Autodesk Fusion 360 part; units mm, degrees
note: some values were not read from the file. Chosen so that the rebuilt part matches the saved one: which pieces of a blend or face edit are solid. Set by a fixed rule: which sketch regions a step uses.
(part 2 of 3)
  line L805 (266.727767, 11.986044) -> (273.65597, -0.013956)
  line L806 (273.65597, -0.013956) -> (287.512376, -0.013956)
  line L807 (287.512376, -0.013956) -> (294.44058, 11.986044)
  line L808 (294.44058, 11.986044) -> (287.512376, 23.986044)
  line L809 (290.110453, 25.486044) -> (297.038656, 13.486044)
  line L810 (297.038656, 37.486044) -> (290.110453, 25.486044)
  line L811 (310.895062, 37.486044) -> (297.038656, 37.486044)
  line L812 (317.823265, 25.486044) -> (310.895062, 37.486044)
  line L813 (310.895062, 13.486044) -> (317.823265, 25.486044)
  line L814 (320.421342, 23.986044) -> (313.493138, 11.986044)
  line L815 (297.038656, 13.486044) -> (310.895062, 13.486044)
  line L816 (310.895062, 10.486044) -> (297.038656, 10.486044)
  line L817 (317.823265, -1.513956) -> (310.895062, 10.486044)
  line L818 (310.895062, -13.513956) -> (317.823265, -1.513956)
  line L819 (297.038656, -13.513956) -> (310.895062, -13.513956)
  line L820 (290.110453, -1.513956) -> (297.038656, -13.513956)
  line L821 (297.038656, 10.486044) -> (290.110453, -1.513956)
  line L822 (334.277748, 23.986044) -> (320.421342, 23.986044)
  line L823 (313.493138, 11.986044) -> (320.421342, -0.013956)
  line L824 (320.421342, -0.013956) -> (334.277748, -0.013956)
  line L825 (334.277748, -0.013956) -> (341.205951, 11.986044)
  line L826 (341.205951, 11.986044) -> (334.277748, 23.986044)
  line L827 (334.277748, -3.013956) -> (320.421342, -3.013956)
  line L828 (320.421342, -3.013956) -> (313.493138, -15.013956)
  line L829 (313.493138, -15.013956) -> (320.421342, -27.013956)
  line L830 (320.421342, -27.013956) -> (334.277748, -27.013956)
  line L831 (334.277748, -27.013956) -> (341.205951, -15.013956)
  line L832 (341.205951, -15.013956) -> (334.277748, -3.013956)
  line L833 (336.875824, -1.513956) -> (343.804028, -13.513956)
  line L834 (343.804028, 10.486044) -> (336.875824, -1.513956)
  line L835 (357.660434, 10.486044) -> (343.804028, 10.486044)
  line L836 (364.588637, -1.513956) -> (357.660434, 10.486044)
  line L837 (357.660434, -13.513956) -> (364.588637, -1.513956)
  line L838 (367.186713, -3.013956) -> (360.25851, -15.013956)
  line L839 (343.804028, -13.513956) -> (357.660434, -13.513956)
  line L840 (357.660434, -16.513956) -> (343.804028, -16.513956)
  line L841 (364.588637, -28.513956) -> (357.660434, -16.513956)
  line L842 (357.660434, -40.513956) -> (364.588637, -28.513956)
  line L843 (343.804028, -40.513956) -> (357.660434, -40.513956)
  line L844 (336.875824, -28.513956) -> (343.804028, -40.513956)
  line L845 (343.804028, -16.513956) -> (336.875824, -28.513956)
  line L846 (381.04312, -3.013956) -> (367.186713, -3.013956)
  line L847 (360.25851, -15.013956) -> (367.186713, -27.013956)
  line L848 (367.186713, -27.013956) -> (381.04312, -27.013956)
  line L849 (381.04312, -27.013956) -> (387.971323, -15.013956)
  line L850 (387.971323, -15.013956) -> (381.04312, -3.013956)
  line L851 (381.04312, -30.013956) -> (367.186713, -30.013956)
  line L852 (367.186713, -30.013956) -> (360.25851, -42.013956)
  line L853 (360.25851, -42.013956) -> (367.186713, -54.013956)
  line L854 (367.186713, -54.013956) -> (381.04312, -54.013956)
  line L855 (381.04312, -54.013956) -> (387.971323, -42.013956)
  line L856 (387.971323, -42.013956) -> (381.04312, -30.013956)
  line L857 (383.641196, -28.513956) -> (390.569399, -40.513956)
  line L858 (390.569399, -16.513956) -> (383.641196, -28.513956)
  line L859 (404.425806, -16.513956) -> (390.569399, -16.513956)
  line L860 (411.354009, -28.513956) -> (404.425806, -16.513956)
  line L861 (404.425806, -40.513956) -> (411.354009, -28.513956)
  line L862 (413.952085, -30.013956) -> (407.023882, -42.013956)
  line L863 (390.569399, -40.513956) -> (404.425806, -40.513956)
  line L864 (404.425806, -43.513956) -> (390.569399, -43.513956)
  line L865 (411.354009, -55.513956) -> (404.425806, -43.513956)
  line L866 (404.425806, -67.513956) -> (411.354009, -55.513956)
  line L867 (390.569399, -67.513956) -> (404.425806, -67.513956)
  line L868 (383.641196, -55.513956) -> (390.569399, -67.513956)
  line L869 (390.569399, -43.513956) -> (383.641196, -55.513956)
  line L870 (427.808492, -30.013956) -> (413.952085, -30.013956)
  line L871 (407.023882, -42.013956) -> (413.952085, -54.013956)
  line L872 (413.952085, -54.013956) -> (427.808492, -54.013956)
  line L873 (427.808492, -54.013956) -> (434.736695, -42.013956)
  line L874 (434.736695, -42.013956) -> (427.808492, -30.013956)
  line L875 (427.808492, -57.013956) -> (413.952085, -57.013956)
  line L876 (413.952085, -57.013956) -> (407.023882, -69.013956)
  line L877 (407.023882, -69.013956) -> (413.952085, -81.013956)
  line L878 (413.952085, -81.013956) -> (427.808492, -81.013956)
  line L879 (427.808492, -81.013956) -> (434.736695, -69.013956)
  line L880 (434.736695, -69.013956) -> (427.808492, -57.013956)
  line L881 (430.406568, -55.513956) -> (437.334771, -67.513956)
  line L882 (437.334771, -43.513956) -> (430.406568, -55.513956)
  line L883 (451.191178, -43.513956) -> (437.334771, -43.513956)
  line L884 (458.119381, -55.513956) -> (451.191178, -43.513956)
  line L885 (451.191178, -67.513956) -> (458.119381, -55.513956)
  line L886 (460.717457, -57.013956) -> (453.789254, -69.013956)
  line L887 (437.334771, -67.513956) -> (451.191178, -67.513956)
  line L888 (451.191178, -70.513956) -> (437.334771, -70.513956)
  line L889 (458.119381, -82.513956) -> (451.191178, -70.513956)
  line L890 (451.191178, -94.513956) -> (458.119381, -82.513956)
  line L891 (437.334771, -94.513956) -> (451.191178, -94.513956)
  line L892 (430.406568, -82.513956) -> (437.334771, -94.513956)
  line L893 (437.334771, -70.513956) -> (430.406568, -82.513956)
  line L894 (474.573864, -57.013956) -> (460.717457, -57.013956)
  line L895 (453.789254, -69.013956) -> (460.717457, -81.013956)
  line L896 (460.717457, -81.013956) -> (474.573864, -81.013956)
  line L897 (474.573864, -81.013956) -> (481.502067, -69.013956)
  line L898 (481.502067, -69.013956) -> (474.573864, -57.013956)
  line L899 (474.573864, -84.013956) -> (460.717457, -84.013956)
  line L900 (460.717457, -84.013956) -> (453.789254, -96.013956)
  line L901 (453.789254, -96.013956) -> (460.717457, -108.013956)
  line L902 (460.717457, -108.013956) -> (474.573864, -108.013956)
  line L903 (474.573864, -108.013956) -> (481.502067, -96.013956)
  line L904 (481.502067, -96.013956) -> (474.573864, -84.013956)
  line L905 (79.663594, 200.981392) -> (86.591797, 188.981392)
  line L906 (86.591797, 212.981392) -> (79.663594, 200.981392)
  line L907 (100.448203, 212.981392) -> (86.591797, 212.981392)
  line L908 (107.376406, 200.981392) -> (100.448203, 212.981392)
  line L909 (100.448203, 188.981392) -> (107.376406, 200.981392)
  line L910 (109.974483, 199.481392) -> (103.046279, 187.481392)
  line L911 (86.591797, 188.981392) -> (100.448203, 188.981392)
  line L912 (100.448203, 185.981392) -> (86.591797, 185.981392)
  line L913 (107.376406, 173.981392) -> (100.448203, 185.981392)
  line L914 (100.448203, 161.981392) -> (107.376406, 173.981392)
  line L915 (86.591797, 161.981392) -> (100.448203, 161.981392)
  line L916 (79.663594, 173.981392) -> (86.591797, 161.981392)
  line L917 (86.591797, 185.981392) -> (79.663594, 173.981392)
  line L918 (123.830889, 199.481392) -> (109.974483, 199.481392)
  line L919 (103.046279, 187.481392) -> (109.974483, 175.481392)
  line L920 (109.974483, 175.481392) -> (123.830889, 175.481392)
  line L921 (123.830889, 175.481392) -> (130.759092, 187.481392)
  line L922 (130.759092, 187.481392) -> (123.830889, 199.481392)
  line L923 (123.830889, 172.481392) -> (109.974483, 172.481392)
  line L924 (109.974483, 172.481392) -> (103.046279, 160.481392)
  line L925 (103.046279, 160.481392) -> (109.974483, 148.481392)
  line L926 (109.974483, 148.481392) -> (123.830889, 148.481392)
  line L927 (123.830889, 148.481392) -> (130.759092, 160.481392)
  line L928 (130.759092, 160.481392) -> (123.830889, 172.481392)
  line L929 (126.428965, 173.981392) -> (133.357169, 161.981392)
  line L930 (133.357169, 185.981392) -> (126.428965, 173.981392)
  line L931 (147.213575, 185.981392) -> (133.357169, 185.981392)
  line L932 (154.141778, 173.981392) -> (147.213575, 185.981392)
  line L933 (147.213575, 161.981392) -> (154.141778, 173.981392)
  line L934 (156.739854, 172.481392) -> (149.811651, 160.481392)
  line L935 (133.357169, 161.981392) -> (147.213575, 161.981392)
  line L936 (147.213575, 158.981392) -> (133.357169, 158.981392)
  line L937 (154.141778, 146.981392) -> (147.213575, 158.981392)
  line L938 (147.213575, 134.981392) -> (154.141778, 146.981392)
  line L939 (133.357169, 134.981392) -> (147.213575, 134.981392)
  line L940 (126.428965, 146.981392) -> (133.357169, 134.981392)
  line L941 (133.357169, 158.981392) -> (126.428965, 146.981392)
  line L942 (170.596261, 172.481392) -> (156.739854, 172.481392)
  line L943 (149.811651, 160.481392) -> (156.739854, 148.481392)
  line L944 (156.739854, 148.481392) -> (170.596261, 148.481392)
  line L945 (170.596261, 148.481392) -> (177.524464, 160.481392)
  line L946 (177.524464, 160.481392) -> (170.596261, 172.481392)
  line L947 (170.596261, 145.481392) -> (156.739854, 145.481392)
  line L948 (156.739854, 145.481392) -> (149.811651, 133.481392)
  line L949 (149.811651, 133.481392) -> (156.739854, 121.481392)
  line L950 (156.739854, 121.481392) -> (170.596261, 121.481392)
  line L951 (170.596261, 121.481392) -> (177.524464, 133.481392)
  line L952 (177.524464, 133.481392) -> (170.596261, 145.481392)
  line L953 (173.194337, 146.981392) -> (180.12254, 134.981392)
  line L954 (180.12254, 158.981392) -> (173.194337, 146.981392)
  line L955 (193.978947, 158.981392) -> (180.12254, 158.981392)
  line L956 (200.90715, 146.981392) -> (193.978947, 158.981392)
  line L957 (193.978947, 134.981392) -> (200.90715, 146.981392)
  line L958 (203.505226, 145.481392) -> (196.577023, 133.481392)
  line L959 (180.12254, 134.981392) -> (193.978947, 134.981392)
  line L960 (193.978947, 131.981392) -> (180.12254, 131.981392)
  line L961 (200.90715, 119.981392) -> (193.978947, 131.981392)
  line L962 (193.978947, 107.981392) -> (200.90715, 119.981392)
  line L963 (180.12254, 107.981392) -> (193.978947, 107.981392)
  line L964 (173.194337, 119.981392) -> (180.12254, 107.981392)
  line L965 (180.12254, 131.981392) -> (173.194337, 119.981392)
  line L966 (217.361633, 145.481392) -> (203.505226, 145.481392)
  line L967 (196.577023, 133.481392) -> (203.505226, 121.481392)
  line L968 (203.505226, 121.481392) -> (217.361633, 121.481392)
  line L969 (217.361633, 121.481392) -> (224.289836, 133.481392)
  line L970 (224.289836, 133.481392) -> (217.361633, 145.481392)
  line L971 (217.361633, 118.481392) -> (203.505226, 118.481392)
  line L972 (203.505226, 118.481392) -> (196.577023, 106.481392)
  line L973 (196.577023, 106.481392) -> (203.505226, 94.481392)
  line L974 (203.505226, 94.481392) -> (217.361633, 94.481392)
  line L975 (217.361633, 94.481392) -> (224.289836, 106.481392)
  line L976 (224.289836, 106.481392) -> (217.361633, 118.481392)
  line L977 (219.959709, 119.981392) -> (226.887912, 107.981392)
  line L978 (226.887912, 131.981392) -> (219.959709, 119.981392)
  line L979 (240.744319, 131.981392) -> (226.887912, 131.981392)
  line L980 (247.672522, 119.981392) -> (240.744319, 131.981392)
  line L981 (240.744319, 107.981392) -> (247.672522, 119.981392)
  line L982 (250.270598, 118.481392) -> (243.342395, 106.481392)
  line L983 (226.887912, 107.981392) -> (240.744319, 107.981392)
  line L984 (240.744319, 104.981392) -> (226.887912, 104.981392)
  line L985 (247.672522, 92.981392) -> (240.744319, 104.981392)
  line L986 (240.744319, 80.981392) -> (247.672522, 92.981392)
  line L987 (226.887912, 80.981392) -> (240.744319, 80.981392)
  line L988 (219.959709, 92.981392) -> (226.887912, 80.981392)
  line L989 (226.887912, 104.981392) -> (219.959709, 92.981392)
  line L990 (264.127005, 118.481392) -> (250.270598, 118.481392)
  line L991 (243.342395, 106.481392) -> (250.270598, 94.481392)
  line L992 (250.270598, 94.481392) -> (264.127005, 94.481392)
  line L993 (264.127005, 94.481392) -> (271.055208, 106.481392)
  line L994 (271.055208, 106.481392) -> (264.127005, 118.481392)
  line L995 (264.127005, 91.481392) -> (250.270598, 91.481392)
  line L996 (250.270598, 91.481392) -> (243.342395, 79.481392)
  line L997 (243.342395, 79.481392) -> (250.270598, 67.481392)
  line L998 (250.270598, 67.481392) -> (264.127005, 67.481392)
  line L999 (264.127005, 67.481392) -> (271.055208, 79.481392)
  line L1000 (271.055208, 79.481392) -> (264.127005, 91.481392)
  line L1001 (266.725081, 92.981392) -> (273.653284, 80.981392)
  line L1002 (273.653284, 104.981392) -> (266.725081, 92.981392)
  line L1003 (287.50969, 104.981392) -> (273.653284, 104.981392)
  line L1004 (294.437894, 92.981392) -> (287.50969, 104.981392)
  line L1005 (287.50969, 80.981392) -> (294.437894, 92.981392)
  line L1006 (297.03597, 91.481392) -> (290.107767, 79.481392)
  line L1007 (273.653284, 80.981392) -> (287.50969, 80.981392)
  line L1008 (287.50969, 77.981392) -> (273.653284, 77.981392)
  line L1009 (294.437894, 65.981392) -> (287.50969, 77.981392)
  line L1010 (287.50969, 53.981392) -> (294.437894, 65.981392)
  line L1011 (273.653284, 53.981392) -> (287.50969, 53.981392)
  line L1012 (266.725081, 65.981392) -> (273.653284, 53.981392)
  line L1013 (273.653284, 77.981392) -> (266.725081, 65.981392)
  line L1014 (310.892376, 91.481392) -> (297.03597, 91.481392)
  line L1015 (290.107767, 79.481392) -> (297.03597, 67.481392)
  line L1016 (297.03597, 67.481392) -> (310.892376, 67.481392)
  line L1017 (310.892376, 67.481392) -> (317.82058, 79.481392)
  line L1018 (317.82058, 79.481392) -> (310.892376, 91.481392)
  line L1019 (310.892376, 64.481392) -> (297.03597, 64.481392)
  line L1020 (297.03597, 64.481392) -> (290.107767, 52.481392)
  line L1021 (290.107767, 52.481392) -> (297.03597, 40.481392)
  line L1022 (297.03597, 40.481392) -> (310.892376, 40.481392)
  line L1023 (310.892376, 40.481392) -> (317.82058, 52.481392)
  line L1024 (317.82058, 52.481392) -> (310.892376, 64.481392)
  line L1025 (313.490453, 65.981392) -> (320.418656, 53.981392)
  line L1026 (320.418656, 77.981392) -> (313.490453, 65.981392)
  line L1027 (334.275062, 77.981392) -> (320.418656, 77.981392)
  line L1028 (341.203265, 65.981392) -> (334.275062, 77.981392)
  line L1029 (334.275062, 53.981392) -> (341.203265, 65.981392)
  line L1030 (343.801342, 64.481392) -> (336.873138, 52.481392)
  line L1031 (320.418656, 53.981392) -> (334.275062, 53.981392)
  line L1032 (334.275062, 50.981392) -> (320.418656, 50.981392)
  line L1033 (341.203265, 38.981392) -> (334.275062, 50.981392)
  line L1034 (334.275062, 26.981392) -> (341.203265, 38.981392)
  line L1035 (320.418656, 26.981392) -> (334.275062, 26.981392)
  line L1036 (313.490453, 38.981392) -> (320.418656, 26.981392)
  line L1037 (320.418656, 50.981392) -> (313.490453, 38.981392)
  line L1038 (357.657748, 64.481392) -> (343.801342, 64.481392)
  line L1039 (336.873138, 52.481392) -> (343.801342, 40.481392)
  line L1040 (343.801342, 40.481392) -> (357.657748, 40.481392)
  line L1041 (357.657748, 40.481392) -> (364.585951, 52.481392)
  line L1042 (364.585951, 52.481392) -> (357.657748, 64.481392)
  line L1043 (357.657748, 37.481392) -> (343.801342, 37.481392)
  line L1044 (343.801342, 37.481392) -> (336.873138, 25.481392)
  line L1045 (336.873138, 25.481392) -> (343.801342, 13.481392)
  line L1046 (343.801342, 13.481392) -> (357.657748, 13.481392)
  line L1047 (357.657748, 13.481392) -> (364.585951, 25.481392)
  line L1048 (364.585951, 25.481392) -> (357.657748, 37.481392)
  line L1049 (360.255824, 38.981392) -> (367.184028, 26.981392)
  line L1050 (367.184028, 50.981392) -> (360.255824, 38.981392)
  line L1051 (381.040434, 50.981392) -> (367.184028, 50.981392)
  line L1052 (387.968637, 38.981392) -> (381.040434, 50.981392)
  line L1053 (381.040434, 26.981392) -> (387.968637, 38.981392)
  line L1054 (390.566713, 37.481392) -> (383.63851, 25.481392)
  line L1055 (367.184028, 26.981392) -> (381.040434, 26.981392)
  line L1056 (381.040434, 23.981392) -> (367.184028, 23.981392)
  line L1057 (387.968637, 11.981392) -> (381.040434, 23.981392)
  line L1058 (381.040434, -0.018608) -> (387.968637, 11.981392)
  line L1059 (367.184028, -0.018608) -> (381.040434, -0.018608)
  line L1060 (360.255824, 11.981392) -> (367.184028, -0.018608)
  line L1061 (367.184028, 23.981392) -> (360.255824, 11.981392)
  line L1062 (404.42312, 37.481392) -> (390.566713, 37.481392)
  line L1063 (383.63851, 25.481392) -> (390.566713, 13.481392)
  line L1064 (390.566713, 13.481392) -> (404.42312, 13.481392)
  line L1065 (404.42312, 13.481392) -> (411.351323, 25.481392)
  line L1066 (411.351323, 25.481392) -> (404.42312, 37.481392)
  line L1067 (404.42312, 10.481392) -> (390.566713, 10.481392)
  line L1068 (390.566713, 10.481392) -> (383.63851, -1.518608)
  line L1069 (383.63851, -1.518608) -> (390.566713, -13.518608)
  line L1070 (390.566713, -13.518608) -> (404.42312, -13.518608)
  line L1071 (404.42312, -13.518608) -> (411.351323, -1.518608)
  line L1072 (411.351323, -1.518608) -> (404.42312, 10.481392)
  line L1073 (407.021196, 11.981392) -> (413.949399, -0.018608)
  line L1074 (413.949399, 23.981392) -> (407.021196, 11.981392)
  line L1075 (427.805806, 23.981392) -> (413.949399, 23.981392)
  line L1076 (434.734009, 11.981392) -> (427.805806, 23.981392)
  line L1077 (427.805806, -0.018608) -> (434.734009, 11.981392)
  line L1078 (437.332085, 10.481392) -> (430.403882, -1.518608)
  line L1079 (413.949399, -0.018608) -> (427.805806, -0.018608)
  line L1080 (427.805806, -3.018608) -> (413.949399, -3.018608)
  line L1081 (434.734009, -15.018608) -> (427.805806, -3.018608)
  line L1082 (427.805806, -27.018608) -> (434.734009, -15.018608)
  line L1083 (413.949399, -27.018608) -> (427.805806, -27.018608)
  line L1084 (407.021196, -15.018608) -> (413.949399, -27.018608)
  line L1085 (413.949399, -3.018608) -> (407.021196, -15.018608)
  line L1086 (451.188492, 10.481392) -> (437.332085, 10.481392)
  line L1087 (430.403882, -1.518608) -> (437.332085, -13.518608)
  line L1088 (437.332085, -13.518608) -> (451.188492, -13.518608)
  line L1089 (451.188492, -13.518608) -> (458.116695, -1.518608)
  line L1090 (458.116695, -1.518608) -> (451.188492, 10.481392)
  line L1091 (451.188492, -16.518608) -> (437.332085, -16.518608)
  line L1092 (437.332085, -16.518608) -> (430.403882, -28.518608)
  line L1093 (430.403882, -28.518608) -> (437.332085, -40.518608)
  line L1094 (437.332085, -40.518608) -> (451.188492, -40.518608)
  line L1095 (451.188492, -40.518608) -> (458.116695, -28.518608)
  line L1096 (458.116695, -28.518608) -> (451.188492, -16.518608)
  line L1097 (453.786568, -15.018608) -> (460.714771, -27.018608)
  line L1098 (460.714771, -3.018608) -> (453.786568, -15.018608)
  line L1099 (474.571178, -3.018608) -> (460.714771, -3.018608)
  line L1100 (481.499381, -15.018608) -> (474.571178, -3.018608)
  line L1101 (474.571178, -27.018608) -> (481.499381, -15.018608)
  line L1102 (484.097457, -16.518608) -> (477.169254, -28.518608)
  line L1103 (460.714771, -27.018608) -> (474.571178, -27.018608)
  line L1104 (474.571178, -30.018608) -> (460.714771, -30.018608)
  line L1105 (481.499381, -42.018608) -> (474.571178, -30.018608)
  line L1106 (474.571178, -54.018608) -> (481.499381, -42.018608)
  line L1107 (460.714771, -54.018608) -> (474.571178, -54.018608)
  line L1108 (453.786568, -42.018608) -> (460.714771, -54.018608)
  line L1109 (460.714771, -30.018608) -> (453.786568, -42.018608)
  line L1110 (497.953864, -16.518608) -> (484.097457, -16.518608)
  line L1111 (477.169254, -28.518608) -> (484.097457, -40.518608)
  line L1112 (484.097457, -40.518608) -> (497.953864, -40.518608)
  line L1113 (497.953864, -40.518608) -> (504.882067, -28.518608)
  line L1114 (504.882067, -28.518608) -> (497.953864, -16.518608)
  line L1115 (497.953864, -43.518608) -> (484.097457, -43.518608)
  line L1116 (484.097457, -43.518608) -> (477.169254, -55.518608)
  line L1117 (477.169254, -55.518608) -> (484.097457, -67.518608)
  line L1118 (484.097457, -67.518608) -> (497.953864, -67.518608)
  line L1119 (497.953864, -67.518608) -> (504.882067, -55.518608)
  line L1120 (504.882067, -55.518608) -> (497.953864, -43.518608)
  line L1121 (103.043594, 241.476739) -> (109.971797, 229.476739)
  line L1122 (109.971797, 253.476739) -> (103.043594, 241.476739)
  line L1123 (123.828203, 253.476739) -> (109.971797, 253.476739)
  line L1124 (130.756406, 241.476739) -> (123.828203, 253.476739)
  line L1125 (123.828203, 229.476739) -> (130.756406, 241.476739)
  line L1126 (133.354483, 239.976739) -> (126.426279, 227.976739)
  line L1127 (109.971797, 229.476739) -> (123.828203, 229.476739)
  line L1128 (123.828203, 226.476739) -> (109.971797, 226.476739)
  line L1129 (130.756406, 214.476739) -> (123.828203, 226.476739)
  line L1130 (123.828203, 202.476739) -> (130.756406, 214.476739)
  line L1131 (109.971797, 202.476739) -> (123.828203, 202.476739)
  line L1132 (103.043594, 214.476739) -> (109.971797, 202.476739)
  line L1133 (109.971797, 226.476739) -> (103.043594, 214.476739)
  line L1134 (147.210889, 239.976739) -> (133.354483, 239.976739)
  line L1135 (126.426279, 227.976739) -> (133.354483, 215.976739)
  line L1136 (133.354483, 215.976739) -> (147.210889, 215.976739)
  line L1137 (147.210889, 215.976739) -> (154.139092, 227.976739)
  line L1138 (154.139092, 227.976739) -> (147.210889, 239.976739)
  line L1139 (147.210889, 212.976739) -> (133.354483, 212.976739)
  line L1140 (133.354483, 212.976739) -> (126.426279, 200.976739)
  line L1141 (126.426279, 200.976739) -> (133.354483, 188.976739)
  line L1142 (133.354483, 188.976739) -> (147.210889, 188.976739)
  line L1143 (147.210889, 188.976739) -> (154.139092, 200.976739)
  line L1144 (154.139092, 200.976739) -> (147.210889, 212.976739)
  line L1145 (149.808965, 214.476739) -> (156.737169, 202.476739)
  line L1146 (156.737169, 226.476739) -> (149.808965, 214.476739)
  line L1147 (170.593575, 226.476739) -> (156.737169, 226.476739)
  line L1148 (177.521778, 214.476739) -> (170.593575, 226.476739)
  line L1149 (170.593575, 202.476739) -> (177.521778, 214.476739)
  line L1150 (180.119854, 212.976739) -> (173.191651, 200.976739)
  line L1151 (156.737169, 202.476739) -> (170.593575, 202.476739)
  line L1152 (170.593575, 199.476739) -> (156.737169, 199.476739)
  line L1153 (177.521778, 187.476739) -> (170.593575, 199.476739)
  line L1154 (170.593575, 175.476739) -> (177.521778, 187.476739)
  line L1155 (156.737169, 175.476739) -> (170.593575, 175.476739)
  line L1156 (149.808965, 187.476739) -> (156.737169, 175.476739)
  line L1157 (156.737169, 199.476739) -> (149.808965, 187.476739)
  line L1158 (193.976261, 212.976739) -> (180.119854, 212.976739)
  line L1159 (173.191651, 200.976739) -> (180.119854, 188.976739)
  line L1160 (180.119854, 188.976739) -> (193.976261, 188.976739)
  line L1161 (193.976261, 188.976739) -> (200.904464, 200.976739)
  line L1162 (200.904464, 200.976739) -> (193.976261, 212.976739)
  line L1163 (193.976261, 185.976739) -> (180.119854, 185.976739)
  line L1164 (180.119854, 185.976739) -> (173.191651, 173.976739)
  line L1165 (173.191651, 173.976739) -> (180.119854, 161.976739)
  line L1166 (180.119854, 161.976739) -> (193.976261, 161.976739)
  line L1167 (193.976261, 161.976739) -> (200.904464, 173.976739)
  line L1168 (200.904464, 173.976739) -> (193.976261, 185.976739)
  line L1169 (196.574337, 187.476739) -> (203.50254, 175.476739)
  line L1170 (203.50254, 199.476739) -> (196.574337, 187.476739)
  line L1171 (217.358947, 199.476739) -> (203.50254, 199.476739)
  line L1172 (224.28715, 187.476739) -> (217.358947, 199.476739)
  line L1173 (217.358947, 175.476739) -> (224.28715, 187.476739)
  line L1174 (226.885226, 185.976739) -> (219.957023, 173.976739)
  line L1175 (203.50254, 175.476739) -> (217.358947, 175.476739)
  line L1176 (217.358947, 172.476739) -> (203.50254, 172.476739)
  line L1177 (224.28715, 160.476739) -> (217.358947, 172.476739)
  line L1178 (217.358947, 148.476739) -> (224.28715, 160.476739)
  line L1179 (203.50254, 148.476739) -> (217.358947, 148.476739)
  line L1180 (196.574337, 160.476739) -> (203.50254, 148.476739)
  line L1181 (203.50254, 172.476739) -> (196.574337, 160.476739)
  line L1182 (240.741633, 185.976739) -> (226.885226, 185.976739)
  line L1183 (219.957023, 173.976739) -> (226.885226, 161.976739)
  line L1184 (226.885226, 161.976739) -> (240.741633, 161.976739)
  line L1185 (240.741633, 161.976739) -> (247.669836, 173.976739)
  line L1186 (247.669836, 173.976739) -> (240.741633, 185.976739)
  line L1187 (240.741633, 158.976739) -> (226.885226, 158.976739)
  line L1188 (226.885226, 158.976739) -> (219.957023, 146.976739)
  line L1189 (219.957023, 146.976739) -> (226.885226, 134.976739)
  line L1190 (226.885226, 134.976739) -> (240.741633, 134.976739)
  line L1191 (240.741633, 134.976739) -> (247.669836, 146.976739)
  line L1192 (247.669836, 146.976739) -> (240.741633, 158.976739)
  line L1193 (243.339709, 160.476739) -> (250.267912, 148.476739)
  line L1194 (250.267912, 172.476739) -> (243.339709, 160.476739)
  line L1195 (264.124319, 172.476739) -> (250.267912, 172.476739)
  line L1196 (271.052522, 160.476739) -> (264.124319, 172.476739)
  line L1197 (264.124319, 148.476739) -> (271.052522, 160.476739)
  line L1198 (273.650598, 158.976739) -> (266.722395, 146.976739)
  line L1199 (250.267912, 148.476739) -> (264.124319, 148.476739)
  line L1200 (264.124319, 145.476739) -> (250.267912, 145.476739)
  line L1201 (271.052522, 133.476739) -> (264.124319, 145.476739)
  line L1202 (264.124319, 121.476739) -> (271.052522, 133.476739)
  line L1203 (250.267912, 121.476739) -> (264.124319, 121.476739)
  line L1204 (243.339709, 133.476739) -> (250.267912, 121.476739)
  line L1205 (250.267912, 145.476739) -> (243.339709, 133.476739)
  line L1206 (287.507005, 158.976739) -> (273.650598, 158.976739)
  line L1207 (266.722395, 146.976739) -> (273.650598, 134.976739)
  line L1208 (273.650598, 134.976739) -> (287.507005, 134.976739)
  line L1209 (287.507005, 134.976739) -> (294.435208, 146.976739)
  line L1210 (294.435208, 146.976739) -> (287.507005, 158.976739)
  line L1211 (287.507005, 131.976739) -> (273.650598, 131.976739)
  line L1212 (273.650598, 131.976739) -> (266.722395, 119.976739)
  line L1213 (266.722395, 119.976739) -> (273.650598, 107.976739)
  line L1214 (273.650598, 107.976739) -> (287.507005, 107.976739)
  line L1215 (287.507005, 107.976739) -> (294.435208, 119.976739)
  line L1216 (294.435208, 119.976739) -> (287.507005, 131.976739)
  line L1217 (290.105081, 133.476739) -> (297.033284, 121.476739)
  line L1218 (297.033284, 145.476739) -> (290.105081, 133.476739)
  line L1219 (310.88969, 145.476739) -> (297.033284, 145.476739)
  line L1220 (317.817894, 133.476739) -> (310.88969, 145.476739)
  line L1221 (310.88969, 121.476739) -> (317.817894, 133.476739)
  line L1222 (320.41597, 131.976739) -> (313.487767, 119.976739)
  line L1223 (297.033284, 121.476739) -> (310.88969, 121.476739)
  line L1224 (310.88969, 118.476739) -> (297.033284, 118.476739)
  line L1225 (317.817894, 106.476739) -> (310.88969, 118.476739)
  line L1226 (310.88969, 94.476739) -> (317.817894, 106.476739)
  line L1227 (297.033284, 94.476739) -> (310.88969, 94.476739)
  line L1228 (290.105081, 106.476739) -> (297.033284, 94.476739)
  line L1229 (297.033284, 118.476739) -> (290.105081, 106.476739)
  line L1230 (334.272376, 131.976739) -> (320.41597, 131.976739)
  line L1231 (313.487767, 119.976739) -> (320.41597, 107.976739)
  line L1232 (320.41597, 107.976739) -> (334.272376, 107.976739)
  line L1233 (334.272376, 107.976739) -> (341.20058, 119.976739)
  line L1234 (341.20058, 119.976739) -> (334.272376, 131.976739)
  line L1235 (334.272376, 104.976739) -> (320.41597, 104.976739)
  line L1236 (320.41597, 104.976739) -> (313.487767, 92.976739)
  line L1237 (313.487767, 92.976739) -> (320.41597, 80.976739)
  line L1238 (320.41597, 80.976739) -> (334.272376, 80.976739)
  line L1239 (334.272376, 80.976739) -> (341.20058, 92.976739)
  line L1240 (341.20058, 92.976739) -> (334.272376, 104.976739)
  line L1241 (336.870453, 106.476739) -> (343.798656, 94.476739)
  line L1242 (343.798656, 118.476739) -> (336.870453, 106.476739)
  line L1243 (357.655062, 118.476739) -> (343.798656, 118.476739)
  line L1244 (364.583265, 106.476739) -> (357.655062, 118.476739)
  line L1245 (357.655062, 94.476739) -> (364.583265, 106.476739)
  line L1246 (367.181342, 104.976739) -> (360.253138, 92.976739)
  line L1247 (343.798656, 94.476739) -> (357.655062, 94.476739)
  line L1248 (357.655062, 91.476739) -> (343.798656, 91.476739)
  line L1249 (364.583265, 79.476739) -> (357.655062, 91.476739)
  line L1250 (357.655062, 67.476739) -> (364.583265, 79.476739)
  line L1251 (343.798656, 67.476739) -> (357.655062, 67.476739)
  line L1252 (336.870453, 79.476739) -> (343.798656, 67.476739)
  line L1253 (343.798656, 91.476739) -> (336.870453, 79.476739)
  line L1254 (381.037748, 104.976739) -> (367.181342, 104.976739)
  line L1255 (360.253138, 92.976739) -> (367.181342, 80.976739)
  line L1256 (367.181342, 80.976739) -> (381.037748, 80.976739)
  line L1257 (381.037748, 80.976739) -> (387.965951, 92.976739)
  line L1258 (387.965951, 92.976739) -> (381.037748, 104.976739)
  line L1259 (381.037748, 77.976739) -> (367.181342, 77.976739)
  line L1260 (367.181342, 77.976739) -> (360.253138, 65.976739)
  line L1261 (360.253138, 65.976739) -> (367.181342, 53.976739)
  line L1262 (367.181342, 53.976739) -> (381.037748, 53.976739)
  line L1263 (381.037748, 53.976739) -> (387.965951, 65.976739)
  line L1264 (387.965951, 65.976739) -> (381.037748, 77.976739)
  line L1265 (383.635824, 79.476739) -> (390.564028, 67.476739)
  line L1266 (390.564028, 91.476739) -> (383.635824, 79.476739)
  line L1267 (404.420434, 91.476739) -> (390.564028, 91.476739)
  line L1268 (411.348637, 79.476739) -> (404.420434, 91.476739)
  line L1269 (404.420434, 67.476739) -> (411.348637, 79.476739)
  line L1270 (413.946713, 77.976739) -> (407.01851, 65.976739)
  line L1271 (390.564028, 67.476739) -> (404.420434, 67.476739)
  line L1272 (404.420434, 64.476739) -> (390.564028, 64.476739)
  line L1273 (411.348637, 52.476739) -> (404.420434, 64.476739)
  line L1274 (404.420434, 40.476739) -> (411.348637, 52.476739)
  line L1275 (390.564028, 40.476739) -> (404.420434, 40.476739)
  line L1276 (383.635824, 52.476739) -> (390.564028, 40.476739)
  line L1277 (390.564028, 64.476739) -> (383.635824, 52.476739)
  line L1278 (427.80312, 77.976739) -> (413.946713, 77.976739)
  line L1279 (407.01851, 65.976739) -> (413.946713, 53.976739)
  line L1280 (413.946713, 53.976739) -> (427.80312, 53.976739)
  line L1281 (427.80312, 53.976739) -> (434.731323, 65.976739)
  line L1282 (434.731323, 65.976739) -> (427.80312, 77.976739)
  line L1283 (427.80312, 50.976739) -> (413.946713, 50.976739)
  line L1284 (413.946713, 50.976739) -> (407.01851, 38.976739)
  line L1285 (407.01851, 38.976739) -> (413.946713, 26.976739)
  line L1286 (413.946713, 26.976739) -> (427.80312, 26.976739)
  line L1287 (427.80312, 26.976739) -> (434.731323, 38.976739)
  line L1288 (434.731323, 38.976739) -> (427.80312, 50.976739)
  line L1289 (430.401196, 52.476739) -> (437.329399, 40.476739)
  line L1290 (437.329399, 64.476739) -> (430.401196, 52.476739)
  line L1291 (451.185806, 64.476739) -> (437.329399, 64.476739)
  line L1292 (458.114009, 52.476739) -> (451.185806, 64.476739)
  line L1293 (451.185806, 40.476739) -> (458.114009, 52.476739)
  line L1294 (460.712085, 50.976739) -> (453.783882, 38.976739)
  line L1295 (437.329399, 40.476739) -> (451.185806, 40.476739)
  line L1296 (451.185806, 37.476739) -> (437.329399, 37.476739)
  line L1297 (458.114009, 25.476739) -> (451.185806, 37.476739)
  line L1298 (451.185806, 13.476739) -> (458.114009, 25.476739)
  line L1299 (437.329399, 13.476739) -> (451.185806, 13.476739)
  line L1300 (430.401196, 25.476739) -> (437.329399, 13.476739)
  line L1301 (437.329399, 37.476739) -> (430.401196, 25.476739)
  line L1302 (474.568492, 50.976739) -> (460.712085, 50.976739)
  line L1303 (453.783882, 38.976739) -> (460.712085, 26.976739)
  line L1304 (460.712085, 26.976739) -> (474.568492, 26.976739)
  line L1305 (474.568492, 26.976739) -> (481.496695, 38.976739)
  line L1306 (481.496695, 38.976739) -> (474.568492, 50.976739)
  line L1307 (474.568492, 23.976739) -> (460.712085, 23.976739)
  line L1308 (460.712085, 23.976739) -> (453.783882, 11.976739)
  line L1309 (453.783882, 11.976739) -> (460.712085, -0.023261)
  line L1310 (460.712085, -0.023261) -> (474.568492, -0.023261)
  line L1311 (474.568492, -0.023261) -> (481.496695, 11.976739)
  line L1312 (481.496695, 11.976739) -> (474.568492, 23.976739)
  line L1313 (477.166568, 25.476739) -> (484.094771, 13.476739)
  line L1314 (484.094771, 37.476739) -> (477.166568, 25.476739)
  line L1315 (497.951178, 37.476739) -> (484.094771, 37.476739)
  line L1316 (504.879381, 25.476739) -> (497.951178, 37.476739)
  line L1317 (497.951178, 13.476739) -> (504.879381, 25.476739)
  line L1318 (507.477457, 23.976739) -> (500.549254, 11.976739)
  line L1319 (484.094771, 13.476739) -> (497.951178, 13.476739)
  line L1320 (497.951178, 10.476739) -> (484.094771, 10.476739)
  line L1321 (504.879381, -1.523261) -> (497.951178, 10.476739)
  line L1322 (497.951178, -13.523261) -> (504.879381, -1.523261)
  line L1323 (484.094771, -13.523261) -> (497.951178, -13.523261)
  line L1324 (477.166568, -1.523261) -> (484.094771, -13.523261)
  line L1325 (484.094771, 10.476739) -> (477.166568, -1.523261)
  line L1326 (521.333864, 23.976739) -> (507.477457, 23.976739)
  line L1327 (500.549254, 11.976739) -> (507.477457, -0.023261)
  line L1328 (507.477457, -0.023261) -> (521.333864, -0.023261)
  line L1329 (521.333864, -0.023261) -> (528.262067, 11.976739)
  line L1330 (528.262067, 11.976739) -> (521.333864, 23.976739)
  line L1331 (521.333864, -3.023261) -> (507.477457, -3.023261)
  line L1332 (507.477457, -3.023261) -> (500.549254, -15.023261)
  line L1333 (500.549254, -15.023261) -> (507.477457, -27.023261)
  line L1334 (507.477457, -27.023261) -> (521.333864, -27.023261)
  line L1335 (521.333864, -27.023261) -> (528.262067, -15.023261)
  line L1336 (528.262067, -15.023261) -> (521.333864, -3.023261)
  line L1337 (126.423594, 281.972087) -> (133.351797, 269.972087)
  line L1338 (133.351797, 293.972087) -> (126.423594, 281.972087)
  line L1339 (147.208203, 293.972087) -> (133.351797, 293.972087)
  line L1340 (154.136406, 281.972087) -> (147.208203, 293.972087)
  line L1341 (147.208203, 269.972087) -> (154.136406, 281.972087)
  line L1342 (156.734483, 280.472087) -> (149.806279, 268.472087)
  line L1343 (133.351797, 269.972087) -> (147.208203, 269.972087)
  line L1344 (147.208203, 266.972087) -> (133.351797, 266.972087)
  line L1345 (154.136406, 254.972087) -> (147.208203, 266.972087)
  line L1346 (147.208203, 242.972087) -> (154.136406, 254.972087)
  line L1347 (133.351797, 242.972087) -> (147.208203, 242.972087)
  line L1348 (126.423594, 254.972087) -> (133.351797, 242.972087)
  line L1349 (133.351797, 266.972087) -> (126.423594, 254.972087)
  line L1350 (170.590889, 280.472087) -> (156.734483, 280.472087)
  line L1351 (149.806279, 268.472087) -> (156.734483, 256.472087)
  line L1352 (156.734483, 256.472087) -> (170.590889, 256.472087)
  line L1353 (170.590889, 256.472087) -> (177.519092, 268.472087)
  line L1354 (177.519092, 268.472087) -> (170.590889, 280.472087)
  line L1355 (170.590889, 253.472087) -> (156.734483, 253.472087)
  line L1356 (156.734483, 253.472087) -> (149.806279, 241.472087)
  line L1357 (149.806279, 241.472087) -> (156.734483, 229.472087)
  line L1358 (156.734483, 229.472087) -> (170.590889, 229.472087)
  line L1359 (170.590889, 229.472087) -> (177.519092, 241.472087)
  line L1360 (177.519092, 241.472087) -> (170.590889, 253.472087)
  line L1361 (173.188965, 254.972087) -> (180.117169, 242.972087)
  line L1362 (180.117169, 266.972087) -> (173.188965, 254.972087)
  line L1363 (193.973575, 266.972087) -> (180.117169, 266.972087)
  line L1364 (200.901778, 254.972087) -> (193.973575, 266.972087)
  line L1365 (193.973575, 242.972087) -> (200.901778, 254.972087)
  line L1366 (203.499854, 253.472087) -> (196.571651, 241.472087)
  line L1367 (180.117169, 242.972087) -> (193.973575, 242.972087)
  line L1368 (193.973575, 239.972087) -> (180.117169, 239.972087)
  line L1369 (200.901778, 227.972087) -> (193.973575, 239.972087)
  line L1370 (193.973575, 215.972087) -> (200.901778, 227.972087)
  line L1371 (180.117169, 215.972087) -> (193.973575, 215.972087)
  line L1372 (173.188965, 227.972087) -> (180.117169, 215.972087)
  line L1373 (180.117169, 239.972087) -> (173.188965, 227.972087)
  line L1374 (217.356261, 253.472087) -> (203.499854, 253.472087)
  line L1375 (196.571651, 241.472087) -> (203.499854, 229.472087)
  line L1376 (203.499854, 229.472087) -> (217.356261, 229.472087)
  line L1377 (217.356261, 229.472087) -> (224.284464, 241.472087)
  line L1378 (224.284464, 241.472087) -> (217.356261, 253.472087)
  line L1379 (217.356261, 226.472087) -> (203.499854, 226.472087)
  line L1380 (203.499854, 226.472087) -> (196.571651, 214.472087)
  line L1381 (196.571651, 214.472087) -> (203.499854, 202.472087)
  line L1382 (203.499854, 202.472087) -> (217.356261, 202.472087)
  line L1383 (217.356261, 202.472087) -> (224.284464, 214.472087)
  line L1384 (224.284464, 214.472087) -> (217.356261, 226.472087)
  line L1385 (219.954337, 227.972087) -> (226.88254, 215.972087)
  line L1386 (226.88254, 239.972087) -> (219.954337, 227.972087)
  line L1387 (240.738947, 239.972087) -> (226.88254, 239.972087)
  line L1388 (247.66715, 227.972087) -> (240.738947, 239.972087)
  line L1389 (240.738947, 215.972087) -> (247.66715, 227.972087)
  line L1390 (250.265226, 226.472087) -> (243.337023, 214.472087)
  line L1391 (226.88254, 215.972087) -> (240.738947, 215.972087)
  line L1392 (240.738947, 212.972087) -> (226.88254, 212.972087)
  line L1393 (247.66715, 200.972087) -> (240.738947, 212.972087)
  line L1394 (240.738947, 188.972087) -> (247.66715, 200.972087)
  line L1395 (226.88254, 188.972087) -> (240.738947, 188.972087)
  line L1396 (219.954337, 200.972087) -> (226.88254, 188.972087)
  line L1397 (226.88254, 212.972087) -> (219.954337, 200.972087)
  line L1398 (264.121633, 226.472087) -> (250.265226, 226.472087)
  line L1399 (243.337023, 214.472087) -> (250.265226, 202.472087)
  line L1400 (250.265226, 202.472087) -> (264.121633, 202.472087)
  line L1401 (264.121633, 202.472087) -> (271.049836, 214.472087)
  line L1402 (271.049836, 214.472087) -> (264.121633, 226.472087)
  line L1403 (264.121633, 199.472087) -> (250.265226, 199.472087)
  line L1404 (250.265226, 199.472087) -> (243.337023, 187.472087)
  line L1405 (243.337023, 187.472087) -> (250.265226, 175.472087)
  line L1406 (250.265226, 175.472087) -> (264.121633, 175.472087)
  line L1407 (264.121633, 175.472087) -> (271.049836, 187.472087)
  line L1408 (271.049836, 187.472087) -> (264.121633, 199.472087)
  line L1409 (266.719709, 200.972087) -> (273.647912, 188.972087)
  line L1410 (273.647912, 212.972087) -> (266.719709, 200.972087)
  line L1411 (287.504319, 212.972087) -> (273.647912, 212.972087)
  line L1412 (294.432522, 200.972087) -> (287.504319, 212.972087)
  line L1413 (287.504319, 188.972087) -> (294.432522, 200.972087)
  line L1414 (297.030598, 199.472087) -> (290.102395, 187.472087)
  line L1415 (273.647912, 188.972087) -> (287.504319, 188.972087)
  line L1416 (287.504319, 185.972087) -> (273.647912, 185.972087)
  line L1417 (294.432522, 173.972087) -> (287.504319, 185.972087)
  line L1418 (287.504319, 161.972087) -> (294.432522, 173.972087)
  line L1419 (273.647912, 161.972087) -> (287.504319, 161.972087)
  line L1420 (266.719709, 173.972087) -> (273.647912, 161.972087)
  line L1421 (273.647912, 185.972087) -> (266.719709, 173.972087)
  line L1422 (310.887005, 199.472087) -> (297.030598, 199.472087)
  line L1423 (290.102395, 187.472087) -> (297.030598, 175.472087)
  line L1424 (297.030598, 175.472087) -> (310.887005, 175.472087)
  line L1425 (310.887005, 175.472087) -> (317.815208, 187.472087)
  line L1426 (317.815208, 187.472087) -> (310.887005, 199.472087)
  line L1427 (310.887005, 172.472087) -> (297.030598, 172.472087)
  line L1428 (297.030598, 172.472087) -> (290.102395, 160.472087)
  line L1429 (290.102395, 160.472087) -> (297.030598, 148.472087)
  line L1430 (297.030598, 148.472087) -> (310.887005, 148.472087)
  line L1431 (310.887005, 148.472087) -> (317.815208, 160.472087)
  line L1432 (317.815208, 160.472087) -> (310.887005, 172.472087)
  line L1433 (313.485081, 173.972087) -> (320.413284, 161.972087)
  line L1434 (320.413284, 185.972087) -> (313.485081, 173.972087)
  line L1435 (334.26969, 185.972087) -> (320.413284, 185.972087)
  line L1436 (341.197894, 173.972087) -> (334.26969, 185.972087)
  line L1437 (334.26969, 161.972087) -> (341.197894, 173.972087)
  line L1438 (343.79597, 172.472087) -> (336.867767, 160.472087)
  line L1439 (320.413284, 161.972087) -> (334.26969, 161.972087)
  line L1440 (334.26969, 158.972087) -> (320.413284, 158.972087)
  line L1441 (341.197894, 146.972087) -> (334.26969, 158.972087)
  line L1442 (334.26969, 134.972087) -> (341.197894, 146.972087)
  line L1443 (320.413284, 134.972087) -> (334.26969, 134.972087)
  line L1444 (313.485081, 146.972087) -> (320.413284, 134.972087)
  line L1445 (320.413284, 158.972087) -> (313.485081, 146.972087)
  line L1446 (357.652376, 172.472087) -> (343.79597, 172.472087)
  line L1447 (336.867767, 160.472087) -> (343.79597, 148.472087)
  line L1448 (343.79597, 148.472087) -> (357.652376, 148.472087)
  line L1449 (357.652376, 148.472087) -> (364.58058, 160.472087)
  line L1450 (364.58058, 160.472087) -> (357.652376, 172.472087)
  line L1451 (357.652376, 145.472087) -> (343.79597, 145.472087)
  line L1452 (343.79597, 145.472087) -> (336.867767, 133.472087)
  line L1453 (336.867767, 133.472087) -> (343.79597, 121.472087)
  line L1454 (343.79597, 121.472087) -> (357.652376, 121.472087)
  line L1455 (357.652376, 121.472087) -> (364.58058, 133.472087)
  line L1456 (364.58058, 133.472087) -> (357.652376, 145.472087)
  line L1457 (360.250453, 146.972087) -> (367.178656, 134.972087)
  line L1458 (367.178656, 158.972087) -> (360.250453, 146.972087)
  line L1459 (381.035062, 158.972087) -> (367.178656, 158.972087)
  line L1460 (387.963265, 146.972087) -> (381.035062, 158.972087)
  line L1461 (381.035062, 134.972087) -> (387.963265, 146.972087)
  line L1462 (390.561342, 145.472087) -> (383.633138, 133.472087)
  line L1463 (367.178656, 134.972087) -> (381.035062, 134.972087)
  line L1464 (381.035062, 131.972087) -> (367.178656, 131.972087)
  line L1465 (387.963265, 119.972087) -> (381.035062, 131.972087)
  line L1466 (381.035062, 107.972087) -> (387.963265, 119.972087)
  line L1467 (367.178656, 107.972087) -> (381.035062, 107.972087)
  line L1468 (360.250453, 119.972087) -> (367.178656, 107.972087)
  line L1469 (367.178656, 131.972087) -> (360.250453, 119.972087)
  line L1470 (404.417748, 145.472087) -> (390.561342, 145.472087)
  line L1471 (383.633138, 133.472087) -> (390.561342, 121.472087)
  line L1472 (390.561342, 121.472087) -> (404.417748, 121.472087)
  line L1473 (404.417748, 121.472087) -> (411.345951, 133.472087)
  line L1474 (411.345951, 133.472087) -> (404.417748, 145.472087)
  line L1475 (404.417748, 118.472087) -> (390.561342, 118.472087)
  line L1476 (390.561342, 118.472087) -> (383.633138, 106.472087)
  line L1477 (383.633138, 106.472087) -> (390.561342, 94.472087)
  line L1478 (390.561342, 94.472087) -> (404.417748, 94.472087)
  line L1479 (404.417748, 94.472087) -> (411.345951, 106.472087)
  line L1480 (411.345951, 106.472087) -> (404.417748, 118.472087)
  line L1481 (407.015824, 119.972087) -> (413.944028, 107.972087)
  line L1482 (413.944028, 131.972087) -> (407.015824, 119.972087)
  line L1483 (427.800434, 131.972087) -> (413.944028, 131.972087)
  line L1484 (434.728637, 119.972087) -> (427.800434, 131.972087)
  line L1485 (427.800434, 107.972087) -> (434.728637, 119.972087)
  line L1486 (437.326713, 118.472087) -> (430.39851, 106.472087)
  line L1487 (413.944028, 107.972087) -> (427.800434, 107.972087)
  line L1488 (427.800434, 104.972087) -> (413.944028, 104.972087)
  line L1489 (434.728637, 92.972087) -> (427.800434, 104.972087)
  line L1490 (427.800434, 80.972087) -> (434.728637, 92.972087)
  line L1491 (413.944028, 80.972087) -> (427.800434, 80.972087)
  line L1492 (407.015824, 92.972087) -> (413.944028, 80.972087)
  line L1493 (413.944028, 104.972087) -> (407.015824, 92.972087)
  line L1494 (451.18312, 118.472087) -> (437.326713, 118.472087)
  line L1495 (430.39851, 106.472087) -> (437.326713, 94.472087)
  line L1496 (437.326713, 94.472087) -> (451.18312, 94.472087)
  line L1497 (451.18312, 94.472087) -> (458.111323, 106.472087)
  line L1498 (458.111323, 106.472087) -> (451.18312, 118.472087)
  line L1499 (451.18312, 91.472087) -> (437.326713, 91.472087)
  line L1500 (437.326713, 91.472087) -> (430.39851, 79.472087)
  line L1501 (430.39851, 79.472087) -> (437.326713, 67.472087)
  line L1502 (437.326713, 67.472087) -> (451.18312, 67.472087)
  line L1503 (451.18312, 67.472087) -> (458.111323, 79.472087)
  line L1504 (458.111323, 79.472087) -> (451.18312, 91.472087)
  line L1505 (453.781196, 92.972087) -> (460.709399, 80.972087)
  line L1506 (460.709399, 104.972087) -> (453.781196, 92.972087)
  line L1507 (474.565806, 104.972087) -> (460.709399, 104.972087)
  line L1508 (481.494009, 92.972087) -> (474.565806, 104.972087)
  line L1509 (474.565806, 80.972087) -> (481.494009, 92.972087)
  line L1510 (484.092085, 91.472087) -> (477.163882, 79.472087)
  line L1511 (460.709399, 80.972087) -> (474.565806, 80.972087)
  line L1512 (474.565806, 77.972087) -> (460.709399, 77.972087)
  line L1513 (481.494009, 65.972087) -> (474.565806, 77.972087)
  line L1514 (474.565806, 53.972087) -> (481.494009, 65.972087)
  line L1515 (460.709399, 53.972087) -> (474.565806, 53.972087)
  line L1516 (453.781196, 65.972087) -> (460.709399, 53.972087)
  line L1517 (460.709399, 77.972087) -> (453.781196, 65.972087)
  line L1518 (497.948492, 91.472087) -> (484.092085, 91.472087)
  line L1519 (477.163882, 79.472087) -> (484.092085, 67.472087)
  line L1520 (484.092085, 67.472087) -> (497.948492, 67.472087)
  line L1521 (497.948492, 67.472087) -> (504.876695, 79.472087)
  line L1522 (504.876695, 79.472087) -> (497.948492, 91.472087)
  line L1523 (497.948492, 64.472087) -> (484.092085, 64.472087)
  line L1524 (484.092085, 64.472087) -> (477.163882, 52.472087)
  line L1525 (477.163882, 52.472087) -> (484.092085, 40.472087)
  line L1526 (484.092085, 40.472087) -> (497.948492, 40.472087)
  line L1527 (497.948492, 40.472087) -> (504.876695, 52.472087)
  line L1528 (504.876695, 52.472087) -> (497.948492, 64.472087)
  line L1529 (500.546568, 65.972087) -> (507.474771, 53.972087)
  line L1530 (507.474771, 77.972087) -> (500.546568, 65.972087)
  line L1531 (521.331178, 77.972087) -> (507.474771, 77.972087)
  line L1532 (528.259381, 65.972087) -> (521.331178, 77.972087)
  line L1533 (521.331178, 53.972087) -> (528.259381, 65.972087)
  line L1534 (530.857457, 64.472087) -> (523.929254, 52.472087)
  line L1535 (507.474771, 53.972087) -> (521.331178, 53.972087)
  line L1536 (521.331178, 50.972087) -> (507.474771, 50.972087)
  line L1537 (528.259381, 38.972087) -> (521.331178, 50.972087)
  line L1538 (521.331178, 26.972087) -> (528.259381, 38.972087)
  line L1539 (507.474771, 26.972087) -> (521.331178, 26.972087)
  line L1540 (500.546568, 38.972087) -> (507.474771, 26.972087)
  line L1541 (507.474771, 50.972087) -> (500.546568, 38.972087)
  line L1542 (544.713864, 64.472087) -> (530.857457, 64.472087)
  line L1543 (523.929254, 52.472087) -> (530.857457, 40.472087)
  line L1544 (530.857457, 40.472087) -> (544.713864, 40.472087)
  line L1545 (544.713864, 40.472087) -> (551.642067, 52.472087)
  line L1546 (551.642067, 52.472087) -> (544.713864, 64.472087)
  line L1547 (544.713864, 37.472087) -> (530.857457, 37.472087)
  line L1548 (530.857457, 37.472087) -> (523.929254, 25.472087)
  line L1549 (523.929254, 25.472087) -> (530.857457, 13.472087)
  line L1550 (530.857457, 13.472087) -> (544.713864, 13.472087)
  line L1551 (544.713864, 13.472087) -> (551.642067, 25.472087)
  line L1552 (551.642067, 25.472087) -> (544.713864, 37.472087)
  line L1553 (349.571343, 81.5) -> (349.226247, 80.947261)
  line L1554 (341.55576, 72.52043) -> (341.05395, 72.230709)
  point P0 (340, 0)
  point P1 (0, 39)
  point P2 (23.382686, 25.5)
  point P3 (0, 12)
  point P4 (23.382686, -1.5)
  point P5 (23.382686, 25.5)
  point P6 (0, 39)
  point P7 (23.382686, 25.5)
  point P8 (0, 12)
  point P9 (23.382686, -1.5)
  point P10 (0, 66)
  dimension "d1" = 490
  dimension "d10" = 20
  dimension "d11" = 20
  dimension "d12" = 20
  dimension "d13" = 20
  dimension "d16" = 4.35
  dimension "d17" = 6
  dimension "d18" = 6
  dimension "d23" = 80
  dimension "d24" = -78
  dimension "d26" = 30
  dimension "d28" = 27
  dimension "d29" = 150
  dimension "d31" = 30
  dimension "d32" = 27
  dimension "d34" = 27
  dimension "d43" = 6
  dimension "d44" = 6
  dimension "d45" = 6
  dimension "d46" = 6
  dimension "d48" = 10
  dimension "d49" = 10
  dimension "d50" = 10
  dimension "d51" = 10
  dimension "d65" = 5
  dimension "d66" = 2.5
  dimension "d67" = 2.5
  dimension "d68" = -2.5
  dimension "d69" = 2.5
  dimension "d70" = 2.5
  dimension "d71" = 2.5
  dimension "d72" = 2.5
  dimension "d78" = 23.382686
  dimension "d79" = 12
  dimension "d80" = 12
  dimension "d81" = 12